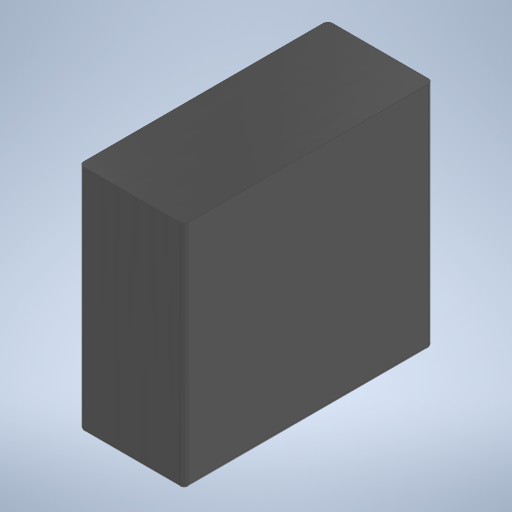
# Autodesk Inventor part: Battery
Saved by Autodesk Inventor 2023 (Build 270158000, 158)
## iProperties
Created: 2022-09-11
Part Number: Battery
Material: Concrete
Document SubType Name: Modeling
Designer: PC
Density: 2.40731 g/cm^3
Appearance: Exposed Aggregate - Coarse
Mass: 2837.29 g
Surface Area: 1856.73 cm^2
Volume: 1178.61 cm^3
Author: PC
Autodesk Inventor part; units mm, degrees
ref_plane "YZ Plane" through (0, 0, 0) normal (1, 0, 0) x (0, 1, 0)
ref_plane "XZ Plane" through (0, 0, 0) normal (0, 1, 0) x (-1, 0, 0)
ref_plane "XY Plane" through (0, 0, 0) normal (0, 0, 1) x (1, 0, 0)
sketch "Sketch1" plane through (0, 0, 0) normal (1, 0, 0) x (0, 1, 0)
  line L0 (0, 0) -> (167.132, 0)
  line L1 (167.132, 0) -> (167.132, -180.34)
  line L2 (167.132, -180.34) -> (0, -180.34)
  line L3 (0, -180.34) -> (0, 0)
  dimension "d0" = 167.132
  dimension "d1" = 180.34
  constraints: 8 end point, 2 parallel, 1 horizontal, 1 perpendicular
  measures "d0" distance of L1.end L2.end
  measures "d1" distance of L0.end L1.end
extrude "Extrusion1" add sketch "Sketch1" along normal blind 76.2
fillet "Fillet1" radius 3.175 8 edges at (76.2, 83.566, 0) (0, 83.566, 0) (76.2, 83.566, -180.34) (0, 83.566, -180.34) (38.1, 0, -180.34) (76.2, 0, -90.17) (38.1, 0, 0) (0, 0, -90.17)
shell "Shell1" thickness 10.16 removed faces 0
body "Solid1"
